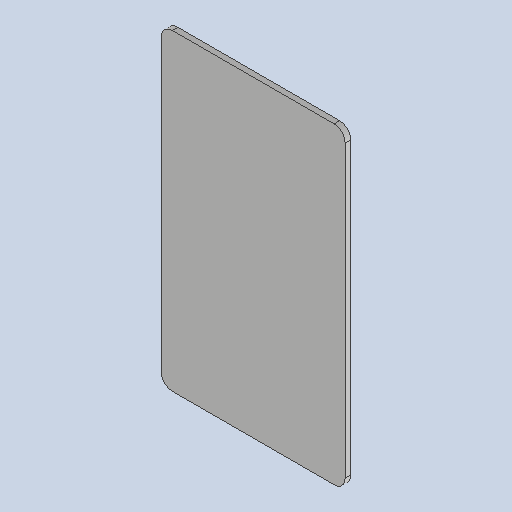
# Autodesk Inventor part: MSC 905 FLANGE BASE TUBE SUPPORT
Saved by Autodesk Inventor 2025 (Build 290162010, 162A)
## iProperties
Created: 2024-07-01
Part Number: MSC 905 FLANGE BASE TUBE SUPPORT
Material: Stainless Steel
Document SubType Name: Sheet Metal
Designer: pokla
Density: 8 g/cm^3
Sheet Metal Rule: AISI304 3mm Die 32
Appearance: Default
Stock Number: МОО 905 опора базовой трубы
Mass: 407.258 g
Surface Area: 355.273 cm^2
Volume: 50.9073 cm^3
Flat Pattern Width: 10 cm
Flat Pattern Length: 17 cm
Flat Pattern Area: 170 cm^2
Sheet Metal Width: 100,000 mm
Sheet Metal Length: 170,000 mm
Sheet Metal Area: 17000,000 mm^2
Author: pokla
Autodesk Inventor part; units mm, degrees
ref_plane "YZ Plane" through (0, 0, 0) normal (1, 0, 0) x (0, 1, 0)
ref_plane "XZ Plane" through (0, 0, 0) normal (0, 1, 0) x (-1, 0, 0)
ref_plane "XY Plane" through (0, 0, 0) normal (0, 0, 1) x (1, 0, 0)
sketch "Sketch1" plane through (0, 0, 0) normal (0, 1, 0) x (-1, 0, 0)
  line L0 (50, 85) -> (-50, 85)
  line L1 (-50, 85) -> (-50, -85)
  line L2 (-50, -85) -> (50, -85)
  line L3 (50, -85) -> (50, 85)
  line L4 (50, 85) -> (-50, -85) construction
  point P0 (0, 0)
  point P1 (0, 0)
  dimension "d0" = 100
  dimension "d1" = 170
  measures "d0" distance of L1.end L2.end
  measures "d1" distance of L0.end L1.end
extrude "Plate1" add sketch "Sketch1" along normal blind 3
fillet "Corner Round1" radius 6 4 edges at (50, 1.5, 85) (-50, 1.5, 85) (50, 1.5, -85) (-50, 1.5, -85)
equation "\"d2\" = Thickness"
equation "\"BendReliefWidth\" = Thickness"
equation "\"BendReliefDepth\" = 0.5 * Thickness"
equation "\"CornerReliefSize\" = 4 * Thickness"
equation "\"MinimumRemnant\" = 2 * Thickness"
equation "\"TransitionRadius\" = BendRadius"
equation "\"JacobiRadiusSize\" = BendRadius"
equation "\"GapSize\" = Thickness"
equation "\"Thickness\" = 3"
equation "\"BendRadius\" = 5"
body "Solid1"
